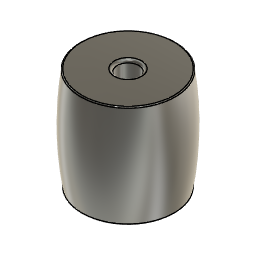
MoldeBalde (Autodesk Fusion 360 archive; units mm, degrees)
design "Borracha_roda"
Autodesk Fusion 360 part; units mm, degrees
sketch "Esboço1" plane through (0, 0, 0) normal (1, 0, 0) x (0, 1, 0)
  line L0 (0, 0) -> (8.5, 0)
  line L1 (0, 0) -> (0, 19)
  line L2 (0, 19) -> (8.7, 19)
  arc A0 (8.5, 0) -> (8.7, 19) centre (-53.1703, 10.1502) ccw
  line L3 (8.5, 0) -> (8.5, 10.6447)
  dimension "d1" = 8.5
  dimension "d2" = 19
  dimension "d3" = 8.7
  dimension "d5" = 125
  constraint coincident L0.start L1.start
  constraint horizontal L0
  constraint perpendicular L0 L1
  constraint perpendicular L1 L2
  constraint perpendicular L0 L3
  measures "d1" distance of L0.start L0.end
  measures "d2" distance of L0.start L1.end
  measures "d3" distance of L1.end L2.end
  measures "d5" diameter of A0
revolve "Revolucionar1" add sketch "Esboço1" angle 360 about axis through (0, 0, 0) along (0, 0, 1)
sketch "Esboço2" plane through (0, 0, 19) normal (0, 0, 1) x (-1, 0, 0)
  circle A0 centre (0, 0) radius 8.7
  circle A1 centre (0, 0) radius 2
  dimension "d7" = 4
  constraint concentric A0 A1
  measures "d7" diameter of A1
extrude "Extrusão1" cut sketch "Esboço2" against normal blind 24 contours A1
fillet "Arredondamento1" radius 0.5 2 edges at (1.8647, -0.7232, 19) (1.8647, 0.7232, 0)
fillet "Arredondamento2" radius 0.2 2 edges at (-8.1112, 3.1461, 19) (-7.9248, 3.0737, 0)
